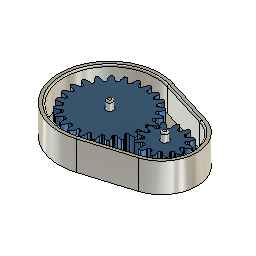
INGRANAGGIO CON GIUNTO v8 (Autodesk Fusion 360 design; units mm, degrees)
description: Spur Gear; Module: 2.000000; Num Teeth: 24; Pressure Angle: 20.000000; Backlash: 0.15 mm
description: Spur Gear; Module: 2.000000; Num Teeth: 12; Pressure Angle: 20.000000; Backlash: 0.15 mm
Autodesk Fusion 360 part; units mm, degrees
note: some values were not read from the file. Set by a fixed rule: which sketch regions a step uses.
sketch "Schizzo1" plane through (0, 0, 0) normal (0, 0, 1) x (1, 0, 0) in component "Spur Gear (24 teeth)"
  circle A0 centre (0, 0) radius 21.5492
  circle A1 centre (0, 0) radius 2.5
extrude "Estrudi1" add sketch "Schizzo1" along normal blind 12.7 makes body 1 in component "Spur Gear (24 teeth)"
sketch "Schizzo2" plane through (0, 0, 0) normal (0, 0, 1) x (1, 0, 0) in component "Spur Gear (24 teeth)"
  spline S0 degree 5 poles (22.4827, -1.7751) (22.4927, -1.7759) (22.5129, -1.7772) (22.5432, -1.7785) (22.5836, -1.7787) (22.6341, -1.777) (22.6847, -1.7739) (22.7353, -1.7699) (22.786, -1.7654) (22.8367, -1.7605) (22.8874, -1.7554) (22.9381, -1.7498) (22.9888, -1.7436) (23.0395, -1.7367) (23.0902, -1.7291) (23.1409, -1.7209) (23.1916, -1.7122) (23.2423, -1.703) (23.2929, -1.6933) (23.3436, -1.6833) (23.3943, -1.673) (23.4449, -1.6622) (23.4956, -1.651) (23.5462, -1.6394) (23.5968, -1.6273) (23.6474, -1.6149) (23.698, -1.602) (23.7486, -1.5888) (23.7991, -1.5752) (23.8497, -1.5613) (23.9002, -1.5471) (23.9506, -1.5325) (24.0011, -1.5175) (24.0515, -1.5022) (24.1019, -1.4866) (24.1523, -1.4706) (24.2027, -1.4543) (24.253, -1.4377) (24.3033, -1.4207) (24.3536, -1.4035) (24.4038, -1.3859) (24.454, -1.368) (24.5042, -1.3499) (24.5543, -1.3314) (24.6044, -1.3126) (24.6545, -1.2935) (24.7045, -1.2742) (24.7546, -1.2545) (24.8045, -1.2346) (24.8545, -1.2143) (24.9044, -1.1938) (24.9542, -1.173) (25.004, -1.1519) (25.0538, -1.1306) (25.1035, -1.109) (25.1532, -1.0871) (25.2029, -1.0649) (25.2525, -1.0425) (25.3021, -1.0198) (25.3516, -0.9968) (25.4011, -0.9736) (25.4505, -0.9501) (25.4999, -0.9263) (25.5493, -0.9023) (25.5986, -0.8781) (25.6478, -0.8535) (25.697, -0.8288) (25.7462, -0.8037) (25.7953, -0.7785) (25.8444, -0.753) (25.8934, -0.7272) (25.9326, -0.7064) (25.9619, -0.6907) (25.9815, -0.6801) (25.9912, -0.6748) knots 0 0 0 0 0 0 0.01428571 0.02857143 0.04285714 0.05714286 0.07142857 0.08571429 0.1 0.11428571 0.12857143 0.14285714 0.15714286 0.17142857 0.18571429 0.2 0.21428571 0.22857143 0.24285714 0.25714286 0.27142857 0.28571429 0.3 0.31428571 0.32857143 0.34285714 0.35714286 0.37142857 0.38571429 0.4 0.41428571 0.42857143 0.44285714 0.45714286 0.47142857 0.48571429 0.5 0.51428571 0.52857143 0.54285714 0.55714286 0.57142857 0.58571429 0.6 0.61428571 0.62857143 0.64285714 0.65714286 0.67142857 0.68571429 0.7 0.71428571 0.72857143 0.74285714 0.75714286 0.77142857 0.78571429 0.8 0.81428571 0.82857143 0.84285714 0.85714286 0.87142857 0.88571429 0.9 0.91428571 0.92857143 0.94285714 0.95714286 0.97142857 0.98571429 1 1 1 1 1 1
  spline S1 degree 5 poles (22.4827, 1.7751) (22.4927, 1.7759) (22.5129, 1.7772) (22.5432, 1.7785) (22.5836, 1.7787) (22.6341, 1.777) (22.6847, 1.7739) (22.7353, 1.7699) (22.786, 1.7654) (22.8367, 1.7605) (22.8874, 1.7554) (22.9381, 1.7498) (22.9888, 1.7436) (23.0395, 1.7367) (23.0902, 1.7291) (23.1409, 1.7209) (23.1916, 1.7122) (23.2423, 1.703) (23.2929, 1.6933) (23.3436, 1.6833) (23.3943, 1.673) (23.4449, 1.6622) (23.4956, 1.651) (23.5462, 1.6394) (23.5968, 1.6273) (23.6474, 1.6149) (23.698, 1.602) (23.7486, 1.5888) (23.7991, 1.5752) (23.8497, 1.5613) (23.9002, 1.5471) (23.9506, 1.5325) (24.0011, 1.5175) (24.0515, 1.5022) (24.1019, 1.4866) (24.1523, 1.4706) (24.2027, 1.4543) (24.253, 1.4377) (24.3033, 1.4207) (24.3536, 1.4035) (24.4038, 1.3859) (24.454, 1.368) (24.5042, 1.3499) (24.5543, 1.3314) (24.6044, 1.3126) (24.6545, 1.2935) (24.7045, 1.2742) (24.7546, 1.2545) (24.8045, 1.2346) (24.8545, 1.2143) (24.9044, 1.1938) (24.9542, 1.173) (25.004, 1.1519) (25.0538, 1.1306) (25.1035, 1.109) (25.1532, 1.0871) (25.2029, 1.0649) (25.2525, 1.0425) (25.3021, 1.0198) (25.3516, 0.9968) (25.4011, 0.9736) (25.4505, 0.9501) (25.4999, 0.9263) (25.5493, 0.9023) (25.5986, 0.8781) (25.6478, 0.8535) (25.697, 0.8288) (25.7462, 0.8037) (25.7953, 0.7785) (25.8444, 0.753) (25.8934, 0.7272) (25.9326, 0.7064) (25.9619, 0.6907) (25.9815, 0.6801) (25.9912, 0.6748) knots 0 0 0 0 0 0 0.01428571 0.02857143 0.04285714 0.05714286 0.07142857 0.08571429 0.1 0.11428571 0.12857143 0.14285714 0.15714286 0.17142857 0.18571429 0.2 0.21428571 0.22857143 0.24285714 0.25714286 0.27142857 0.28571429 0.3 0.31428571 0.32857143 0.34285714 0.35714286 0.37142857 0.38571429 0.4 0.41428571 0.42857143 0.44285714 0.45714286 0.47142857 0.48571429 0.5 0.51428571 0.52857143 0.54285714 0.55714286 0.57142857 0.58571429 0.6 0.61428571 0.62857143 0.64285714 0.65714286 0.67142857 0.68571429 0.7 0.71428571 0.72857143 0.74285714 0.75714286 0.77142857 0.78571429 0.8 0.81428571 0.82857143 0.84285714 0.85714286 0.87142857 0.88571429 0.9 0.91428571 0.92857143 0.94285714 0.95714286 0.97142857 0.98571429 1 1 1 1 1 1
  arc A0 (25.9912, -0.6748) -> (25.9912, 0.6748) centre (0, 0) ccw
  line L0 (21.4724, -1.6961) -> (22.4827, -1.7751)
  line L1 (21.4724, 1.6961) -> (22.4827, 1.7751)
  line L2 (21.4724, -1.6961) -> (21.4724, 1.6961)
  point P0 (22.73, -1.7702)
  point P1 (22.979, -1.7447)
  point P2 (23.2288, -1.7053)
  point P3 (23.4794, -1.6545)
  point P4 (23.7304, -1.5935)
  point P5 (23.9817, -1.5232)
  point P6 (24.2333, -1.4441)
  point P7 (24.485, -1.3568)
  point P8 (24.7366, -1.2615)
  point P9 (24.9882, -1.1586)
  point P10 (25.2395, -1.0483)
  point P11 (25.4905, -0.9308)
  point P12 (25.7411, -0.8063)
  point P13 (22.73, 1.7702)
  point P14 (22.979, 1.7447)
  point P15 (23.2288, 1.7053)
  point P16 (23.4794, 1.6545)
  point P17 (23.7304, 1.5935)
  point P18 (23.9817, 1.5232)
  point P19 (24.2333, 1.4441)
  point P20 (24.485, 1.3568)
  point P21 (24.7366, 1.2615)
  point P22 (24.9882, 1.1586)
  point P23 (25.2395, 1.0483)
  point P24 (25.4905, 0.9308)
  point P25 (25.7411, 0.8063)
extrude "Estrudi2" add sketch "Schizzo2" along normal blind 12.7 bodies 1 in component "Spur Gear (24 teeth)"
fillet "Raccordo1" radius 1 2 edges at (21.4823, -1.6969, 6.35) (21.4823, 1.6969, 6.35) on bodies 1 in component "Spur Gear (24 teeth)"
pattern_circular "Serie C1" count 24 over 360 about axis through (0, 0, 0) along (0, 0, 1) of "Estrudi2", "Raccordo1" in component "Spur Gear (24 teeth)"
sketch "Schizzo3" plane through (0, 0, 0) normal (0, 0, 1) x (1, 0, 0) in component "Spur Gear (24 teeth)"
  circle A0 centre (0, 0) radius 24 construction
sketch "Schizzo1 (2)" plane through (0, 0, 0) normal (0, 0, 1) x (1, 0, 0) in component "Spur Gear (12 teeth)"
  circle A0 centre (0, 0) radius 9.5492
  circle A1 centre (0, 0) radius 2.5
extrude "Estrudi1'" add sketch "Schizzo1 (2)" along normal blind 12.7 separate body makes body 2 in component "Spur Gear (12 teeth)"
sketch "Schizzo2 (2)" plane through (0, 0, 0) normal (0, 0, 1) x (1, 0, 0) in component "Spur Gear (12 teeth)"
  spline S0 degree 5 poles (11.1617, -1.6034) (11.1697, -1.6046) (11.1857, -1.6066) (11.2098, -1.6089) (11.2421, -1.6105) (11.2825, -1.6105) (11.3231, -1.6091) (11.3637, -1.6068) (11.4044, -1.604) (11.4452, -1.6009) (11.486, -1.5974) (11.5268, -1.5934) (11.5676, -1.5889) (11.6085, -1.5836) (11.6494, -1.5776) (11.6904, -1.571) (11.7313, -1.5638) (11.7723, -1.5561) (11.8133, -1.548) (11.8543, -1.5396) (11.8953, -1.5307) (11.9363, -1.5214) (11.9773, -1.5116) (12.0183, -1.5014) (12.0593, -1.4908) (12.1003, -1.4797) (12.1412, -1.4682) (12.1822, -1.4564) (12.2231, -1.4441) (12.2641, -1.4315) (12.305, -1.4185) (12.3459, -1.4051) (12.3868, -1.3914) (12.4276, -1.3773) (12.4685, -1.3628) (12.5093, -1.348) (12.5501, -1.3328) (12.5908, -1.3173) (12.6315, -1.3014) (12.6722, -1.2852) (12.7129, -1.2687) (12.7535, -1.2518) (12.7941, -1.2347) (12.8346, -1.2171) (12.8751, -1.1993) (12.9156, -1.1811) (12.956, -1.1626) (12.9964, -1.1438) (13.0368, -1.1247) (13.077, -1.1053) (13.1173, -1.0855) (13.1575, -1.0655) (13.1976, -1.0451) (13.2377, -1.0245) (13.2778, -1.0035) (13.3178, -0.9822) (13.3577, -0.9607) (13.3976, -0.9389) (13.4374, -0.9167) (13.4771, -0.8943) (13.5168, -0.8716) (13.5565, -0.8486) (13.5961, -0.8253) (13.6356, -0.8017) (13.675, -0.7779) (13.7144, -0.7537) (13.7537, -0.7293) (13.793, -0.7046) (13.8321, -0.6796) (13.8712, -0.6544) (13.9103, -0.6289) (13.9414, -0.6083) (13.9648, -0.5927) (13.9803, -0.5822) (13.9881, -0.577) knots 0 0 0 0 0 0 0.01428571 0.02857143 0.04285714 0.05714286 0.07142857 0.08571429 0.1 0.11428571 0.12857143 0.14285714 0.15714286 0.17142857 0.18571429 0.2 0.21428571 0.22857143 0.24285714 0.25714286 0.27142857 0.28571429 0.3 0.31428571 0.32857143 0.34285714 0.35714286 0.37142857 0.38571429 0.4 0.41428571 0.42857143 0.44285714 0.45714286 0.47142857 0.48571429 0.5 0.51428571 0.52857143 0.54285714 0.55714286 0.57142857 0.58571429 0.6 0.61428571 0.62857143 0.64285714 0.65714286 0.67142857 0.68571429 0.7 0.71428571 0.72857143 0.74285714 0.75714286 0.77142857 0.78571429 0.8 0.81428571 0.82857143 0.84285714 0.85714286 0.87142857 0.88571429 0.9 0.91428571 0.92857143 0.94285714 0.95714286 0.97142857 0.98571429 1 1 1 1 1 1
  spline S1 degree 5 poles (11.1617, 1.6034) (11.1697, 1.6046) (11.1857, 1.6066) (11.2098, 1.6089) (11.2421, 1.6105) (11.2825, 1.6105) (11.3231, 1.6091) (11.3637, 1.6068) (11.4044, 1.604) (11.4452, 1.6009) (11.486, 1.5974) (11.5268, 1.5934) (11.5676, 1.5889) (11.6085, 1.5836) (11.6494, 1.5776) (11.6904, 1.571) (11.7313, 1.5638) (11.7723, 1.5561) (11.8133, 1.548) (11.8543, 1.5396) (11.8953, 1.5307) (11.9363, 1.5214) (11.9773, 1.5116) (12.0183, 1.5014) (12.0593, 1.4908) (12.1003, 1.4797) (12.1412, 1.4682) (12.1822, 1.4564) (12.2231, 1.4441) (12.2641, 1.4315) (12.305, 1.4185) (12.3459, 1.4051) (12.3868, 1.3914) (12.4276, 1.3773) (12.4685, 1.3628) (12.5093, 1.348) (12.5501, 1.3328) (12.5908, 1.3173) (12.6315, 1.3014) (12.6722, 1.2852) (12.7129, 1.2687) (12.7535, 1.2518) (12.7941, 1.2347) (12.8346, 1.2171) (12.8751, 1.1993) (12.9156, 1.1811) (12.956, 1.1626) (12.9964, 1.1438) (13.0368, 1.1247) (13.077, 1.1053) (13.1173, 1.0855) (13.1575, 1.0655) (13.1976, 1.0451) (13.2377, 1.0245) (13.2778, 1.0035) (13.3178, 0.9822) (13.3577, 0.9607) (13.3976, 0.9389) (13.4374, 0.9167) (13.4771, 0.8943) (13.5168, 0.8716) (13.5565, 0.8486) (13.5961, 0.8253) (13.6356, 0.8017) (13.675, 0.7779) (13.7144, 0.7537) (13.7537, 0.7293) (13.793, 0.7046) (13.8321, 0.6796) (13.8712, 0.6544) (13.9103, 0.6289) (13.9414, 0.6083) (13.9648, 0.5927) (13.9803, 0.5822) (13.9881, 0.577) knots 0 0 0 0 0 0 0.01428571 0.02857143 0.04285714 0.05714286 0.07142857 0.08571429 0.1 0.11428571 0.12857143 0.14285714 0.15714286 0.17142857 0.18571429 0.2 0.21428571 0.22857143 0.24285714 0.25714286 0.27142857 0.28571429 0.3 0.31428571 0.32857143 0.34285714 0.35714286 0.37142857 0.38571429 0.4 0.41428571 0.42857143 0.44285714 0.45714286 0.47142857 0.48571429 0.5 0.51428571 0.52857143 0.54285714 0.55714286 0.57142857 0.58571429 0.6 0.61428571 0.62857143 0.64285714 0.65714286 0.67142857 0.68571429 0.7 0.71428571 0.72857143 0.74285714 0.75714286 0.77142857 0.78571429 0.8 0.81428571 0.82857143 0.84285714 0.85714286 0.87142857 0.88571429 0.9 0.91428571 0.92857143 0.94285714 0.95714286 0.97142857 0.98571429 1 1 1 1 1 1
  arc A0 (13.9881, -0.577) -> (13.9881, 0.577) centre (0, 0) ccw
  line L0 (9.4423, -1.3579) -> (11.1617, -1.6034)
  line L1 (9.4423, 1.3579) -> (11.1617, 1.6034)
  line L2 (9.4423, -1.3579) -> (9.4423, 1.3579)
  point P0 (11.3577, -1.607)
  point P1 (11.5565, -1.59)
  point P2 (11.7571, -1.5589)
  point P3 (11.9588, -1.516)
  point P4 (12.1615, -1.4623)
  point P5 (12.3647, -1.3987)
  point P6 (12.5684, -1.3258)
  point P7 (12.7723, -1.2438)
  point P8 (12.9761, -1.1532)
  point P9 (13.1797, -1.0542)
  point P10 (13.3829, -0.9468)
  point P11 (13.5855, -0.8315)
  point P12 (13.7873, -0.7081)
  point P13 (11.3577, 1.607)
  point P14 (11.5565, 1.59)
  point P15 (11.7571, 1.5589)
  point P16 (11.9588, 1.516)
  point P17 (12.1615, 1.4623)
  point P18 (12.3647, 1.3987)
  point P19 (12.5684, 1.3258)
  point P20 (12.7723, 1.2438)
  point P21 (12.9761, 1.1532)
  point P22 (13.1797, 1.0542)
  point P23 (13.3829, 0.9468)
  point P24 (13.5855, 0.8315)
  point P25 (13.7873, 0.7081)
extrude "Estrudi2'" add sketch "Schizzo2 (2)" along normal blind 12.7 bodies 2 in component "Spur Gear (12 teeth)"
fillet "Raccordo1'" radius 1 2 edges at (9.452, -1.3592, 6.35) (9.452, 1.3592, 6.35) on bodies 2 in component "Spur Gear (12 teeth)"
pattern_circular "Serie C1'" count 12 over 360 about axis through (0, 0, 0) along (0, 0, 1) of "Estrudi2'", "Raccordo1'" in component "Spur Gear (12 teeth)"
sketch "Schizzo3 (2)" plane through (0, 0, 0) normal (0, 0, 1) x (1, 0, 0) in component "Spur Gear (12 teeth)"
  circle A0 centre (0, 0) radius 12 construction
move_body "Sposta1" bodies 2 to x (0.965926, 0.258819, 0) y (-0.258819, 0.965926, 0) z (0, 0, 1) at (0, 0, 0) in component "Spur Gear (12 teeth)"
move_body "Sposta2" bodies 2 to x (1, 0, 0) y (0, 1, 0) z (0, 0, 1) at (-1, 0, 0) in component "Spur Gear (12 teeth)"
sketch "Schizzo1 (3)" plane through (0, 0, 0) normal (0, 0, 1) x (1, 0, 0)
  circle A0 centre (0, 0) radius 30
  circle A1 centre (33.9467, -0.0175) radius 20
  line L0 (-5.5131, 33.1006) -> (62.4869, 12.1006)
  line L1 (-6.7774, -33.4734) -> (58.2226, -13.4734)
  dimension "d18" = 60
  dimension "d19" = 40
  constraint coincident A0.centre origin
  constraint tangent A0 L0
  constraint tangent A0 L1
  constraint tangent A1 L0
  constraint tangent A1 L1
  measures "d18" diameter of A0
  measures "d19" diameter of A1
extrude "Estrudi1''" add sketch "Schizzo1 (3)" along normal blind 16 separate body makes body 3
shell "Shell1" thickness 3 outward yes removed faces 1 at (19.1677, -6.3807, 16) on bodies 3
sketch "Schizzo2 (3)" plane through (0, 0, 0) normal (0, 0, 1) x (1, 0, 0)
  circle A0 centre (0, 0) radius 2
  circle A1 centre (36, 0) radius 2
  dimension "d23" = 4
  constraint coincident A0.centre origin
  measures "d23" diameter of A1
extrude "Estrudi2''" add sketch "Schizzo2 (3)" along normal blind 18 bodies 3
fillet "Fillet1" radius 1 2 edges at (-1.8647, -0.7232, 18) (34.1353, -0.7232, 18) on bodies 3
fillet "Fillet2" radius 1 4 edges at (53.9467, -0.0278, 16) (24.3256, -23.9032, 16) (-30, 0.0153, 16) (24.3501, 23.8781, 16) on bodies 3
component "Spur Gear (24 teeth)" placed x (1, 0, 0) y (0, 1, 0) z (0, 0, 1) at (0, 0, 0)
component "Spur Gear (12 teeth)" placed x (1, 0, 0) y (0, 1, 0) z (0, 0, 1) at (37, 0, 0)
component "Base" placed x (1, 0, 0) y (0, 1, 0) z (0, 0, 1) at (0, 0, 0)
equation "taperAngle1 = 0.0 deg"
equation "Radius = 1.00 mm"
equation "countU = 24"
